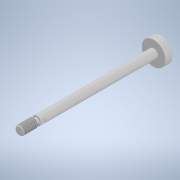
# Autodesk Inventor part: 4186566 DPDM-Q-50---(r)
Saved by Autodesk Inventor 2021 (Build 250183000, 183)
## iProperties
Created: 2026-04-25
Part Number: 4186566 DPDM-Q-50---(r)
Material: Generic
Catalog Web Link: www.3dfindit.com
Description: DPDM(r)-Piston rod
Vendor: FESTO
Document SubType Name: Modeling
Designer: psAdmin
Manufacturer: FESTO
Mass: 3.55207 g
Surface Area: 23.7808 cm^2
Volume: 3.55207 cm^3
Density: 1 g/cm^3
Appearance: PSOLRGB-176-176-176
Category: PARTsolutions
Company: FESTO
Title: 4186566 DPDM-Q-50---(r)
Author: Cadenas PARTsolutions
Comments: Piston rod
PSOL_IDENT_0: {$CADENAS_DATA/23d-libs/festo/parts/d/dpdm/parts/dpdm_rod.prj},205 {VTYP=3D},{NB=4186566 DPDM-Q-50--
PSOL_IDENT_1: -(r)},{LINA=4186566 DPDM-Q-50---(r)},{NN=DPDM(r)},{DATE=23.02.2024 08:53:25},{GEOMDATE=23.02.2024 08
PSOL_IDENT_2: :53:25},{VERSION=},{LINEID=30},{WBVAR=VER,HUB,FUN,KOT},{WBNUMERIC=HUB}  {NB=4186566 DPDM-Q-50---(r)}
PSOL_IDENT_3: ,{LINA=4186566 DPDM-Q-50---(r)},{KT=DUMMY},{TNR=4186566},{TYP=DPDM},{KOL=16},{VER=Q},{VERNB=-Q},{HUB=
PSOL_IDENT_4: 50},{HUB1=5,10,15,20,25,30,40,50},{FUN=-},{FUN1='-'},{FUNNB=},{KOT=-},{KOT1='-','H','T'},{KOTNB=},{A
PSOL_IDENT_5: M=12.000},{KK=M6},{KKN=6.000},{WH=5.000},{MM=6.000},{SW=5.000},{LS=3.000},{ZJ=45.000},{ZM=50.000},{W
PSOL_IDENT_6: 22=3.000},{L2=40.000},{L4=52.000},{L5=12.000},{L6=3.000},{L8=57.000},{L1=22.6},{D8=2.300},{L9=7.000}
NB: 4186566 DPDM-Q-50---(r)
NN: DPDM(r)
NT: Pirston rod
NBSYN: $TNR. $TYP.$VERNB.-$HUB.$FUNNB.$KOTNB.---(r)
LINA: 4186566 DPDM-Q-50---(r)
CATALOG: Festo
TNR: 4186566
TYP: DPDM
KOL: 16
VER: Q
HUB: 50
FUN: -
KOT: -
AM: 12
KK: M6
KKN: 6
WH: 5
MM: 6
SW: 5
LS: 3
ZJ: 45
ZM: 50
W22: 3
L2: 40
L4: 52
L5: 12
L6: 3
L8: 57
D8: 2.3
L9: 7
SUPPLIER: FESTO
ARTICLENO: 4186566 DPDM-Q-50---(r)
BOMINFO: 4186566 DPDM-Q-50---(r)
CREATOR: CADENAS GmbH
Autodesk Inventor part; units mm, degrees
sketch "Sketch_1" plane through (0, 0, 0) normal (1, 0, 0) x (0, 1, 0)
  line L0 (0, -84.4) -> (0, 0)
  line L1 (0, 0) -> (3, 0)
  line L2 (3, 0) -> (3, -79.4)
  line L3 (3, -79.4) -> (8, -79.4)
  line L4 (8, -79.4) -> (8, -84.4)
  line L5 (8, -84.4) -> (0, -84.4)
  line L6 (0, -84.4) -> (0, 0)
  constraints: 14 end point
revolve "Revolution1" add sketch "Sketch_1" angle 360 about axis through (0, 0, -84.4) along (0, 0, -1)
sketch "Sketch_2" plane through (0, 0, 0) normal (1, 0, 0) x (0, 1, 0)
  line L0 (0, 0) -> (0, 12)
  line L1 (0, 12) -> (2.3865, 12)
  line L2 (2.3865, 12) -> (3, 11.3865)
  line L3 (3, 11.3865) -> (3, 2.2222)
  line L4 (3, 2.2222) -> (2.0586, 1.2808)
  arc A0 (2.0586, 1.2808) -> (2, 1.1394) centre (2.2, 1.1394) ccw
  line L5 (2, 1.1394) -> (2, 0.2)
  arc A1 (2, 0.2) -> (2.2, 0) centre (2.2, 0.2) ccw
  line L6 (2.2, 0) -> (0, 0)
  line L7 (0, 0) -> (0, 12)
  constraints: 16 end point, 4 point on circle, 2 centre point
revolve "Revolution2" add sketch "Sketch_2" angle 360 about axis through (0, 0, 0) along (0, 0, -1)
thread "Thread1" size "M6x1" class "6g" standard "ISO Metric profile" full length
sketch "Sketch_8" plane through (0, 0, 0) normal (0, 0, 1) x (1, 0, 0)
  line L0 (-4.5, 5) -> (-4.5, -5)
  line L1 (-4.5, -5) -> (4.5, -5)
  line L2 (4.5, -5) -> (4.5, 5)
  line L3 (4.5, 5) -> (-4.5, 5)
  line L4 (-2.5, -4) -> (2.5, -4)
  line L5 (2.5, -4) -> (2.5, 4)
  line L6 (2.5, 4) -> (-2.5, 4)
  line L7 (-2.5, 4) -> (-2.5, -4)
  constraints: 16 end point
extrude "Extrusion1" cut sketch "Sketch_8" against normal blind 3
ref_plane "CP1_XY" through (0, 0, -84.4) normal (0, 0, -1) x (1, 0, 0)
ref_plane "CP1_YZ" through (0, 0, -84.4) normal (1, 0, 0) x (0, -1, 0)
ref_plane "CP1_ZX" through (0, 0, -84.4) normal (0, -1, 0) x (0, 0, -1)
ref_plane "CP_P_XY" through (0, 0, -84.4) normal (0, 0, 1) x (1, 0, 0)
ref_plane "CP_P_YZ" through (0, 0, -84.4) normal (1, 0, 0) x (0, 1, 0)
ref_plane "CP_P_ZX" through (0, 0, -84.4) normal (0, 1, 0) x (0, 0, 1)
ref_plane "CP_PL_XY" through (0, 0, -3) normal (0, 0, 1) x (1, 0, 0)
ref_plane "CP_PL_YZ" through (0, 0, -3) normal (1, 0, 0) x (0, 1, 0)
ref_plane "CP_PL_ZX" through (0, 0, -3) normal (0, 1, 0) x (0, 0, 1)
ref_plane "DIM_ZM_XY" through (0, 3, -157) normal (1, 0, 0) x (0, 0, -1)
ref_plane "DIM_ZM_YZ" through (0, 3, -157) normal (0, 0, -1) x (0, 1, 0)
ref_plane "DIM_ZM_ZX" through (0, 3, -157) normal (0, 1, 0) x (1, 0, 0)
ref_plane "DISC_XY" through (0, 0, 5) normal (0, 0, -1) x (1, 0, 0)
ref_plane "DISC_YZ" through (0, 0, 5) normal (1, 0, 0) x (0, -1, 0)
ref_plane "DISC_ZX" through (0, 0, 5) normal (0, -1, 0) x (0, 0, -1)
ref_plane "NUT_6_10_T_1_XY" through (0, 0, -168) normal (0, 0, 1) x (1, 0, 0)
ref_plane "NUT_6_10_T_1_YZ" through (0, 0, -168) normal (1, 0, 0) x (0, 1, 0)
ref_plane "NUT_6_10_T_1_ZX" through (0, 0, -168) normal (0, 1, 0) x (0, 0, 1)
ref_plane "NUT_6_10_T_2_XY" through (0, 0, -165.8) normal (0, 0, 1) x (1, 0, 0)
ref_plane "NUT_6_10_T_2_YZ" through (0, 0, -165.8) normal (1, 0, 0) x (0, 1, 0)
ref_plane "NUT_6_10_T_2_ZX" through (0, 0, -165.8) normal (0, 1, 0) x (0, 0, 1)
ref_plane "NUT_CP_6_10_1_XY" through (0, 0, 10) normal (0, 0, 1) x (1, 0, 0)
ref_plane "NUT_CP_6_10_1_YZ" through (0, 0, 10) normal (1, 0, 0) x (0, 1, 0)
ref_plane "NUT_CP_6_10_1_ZX" through (0, 0, 10) normal (0, 1, 0) x (0, 0, 1)
ref_plane "NUT_CP_6_10_2_XY" through (0, 0, 7.8) normal (0, 0, 1) x (1, 0, 0)
ref_plane "NUT_CP_6_10_2_YZ" through (0, 0, 7.8) normal (1, 0, 0) x (0, 1, 0)
ref_plane "NUT_CP_6_10_2_ZX" through (0, 0, 7.8) normal (0, 1, 0) x (0, 0, 1)
body "Solid1"
